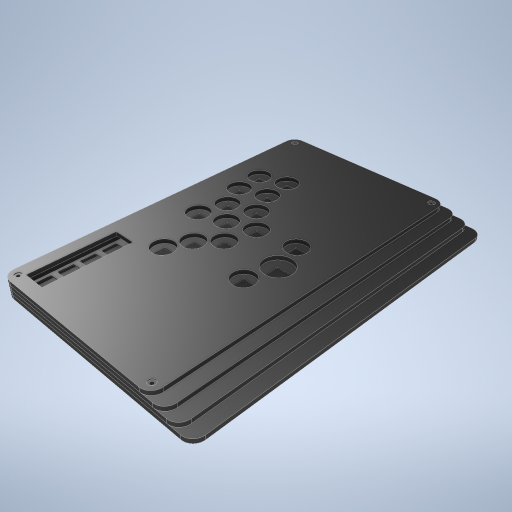
# Autodesk Inventor part: frame
Saved by Autodesk Inventor 2024 (Build 280153000, 153)
## iProperties
Created: 2023-10-17
Part Number: frame
Material: 玻璃
Document SubType Name: Modeling
Designer: Administrator
Density: 2.18 g/cm^3
Appearance: 有光泽 - 黑色
Author: Administrator
Autodesk Inventor part; units mm, degrees
ref_plane "YZ Plane" through (0, 0, 0) normal (1, 0, 0) x (0, 1, 0)
ref_plane "XY Plane" through (0, 0, 0) normal (0, 0, 1) x (1, 0, 0)
ref_plane "底层" through (0, -2, 0) normal (0, 1, 0) x (-1, 0, 0)
ref_plane "第二层" through (0, 4, 0) normal (0, 1, 0) x (-1, 0, 0)
ref_plane "第三层" through (0, 8, 0) normal (0, 1, 0) x (-1, 0, 0)
ref_plane "第四层" through (0, 12, 0) normal (0, 1, 0) x (-1, 0, 0)
sketch "第一层草图" plane through (0, 0, 0) normal (0, 1, 0) x (-1, 0, 0)
  line L0 (90, 150) -> (-90, 150)
  line L1 (-100, 140) -> (-100, -140)
  line L2 (-90, -150) -> (90, -150)
  line L3 (100, -140) -> (100, 140)
  line L4 (100, 150) -> (-100, -150) construction
  line L5 (-100, 150) -> (100, -150) construction
  arc A0 (100, 140) -> (90, 150) centre (90, 140) ccw
  arc A1 (-90, 150) -> (-100, 140) centre (-90, 140) ccw
  arc A2 (-100, -140) -> (-90, -150) centre (-90, -140) ccw
  arc A3 (90, -150) -> (100, -140) centre (90, -140) ccw
  point P0 (0, 0)
  dimension "d2" = 200
  dimension "d3" = 300
  dimension "d4" = 10
  constraints: 12 end point, 8 point on circle, 8 point on line, 8 tangent, 4 centre point, 3 equal radius, 2 midpoint, 2 parallel, 1 horizontal, 1 perpendicular
  measures "d2" distance of L5.end L4.end
  measures "d3" distance of L4.end L5.start
  measures "d4" radius of A0
sketch "第二层草图" plane through (0, 4, 0) normal (0, 1, 0) x (-1, 0, 0)
  line L0 (100, -140) -> (100, 140) projected
  line L1 (100, 0) -> (-88, 0)
  line L2 (90, 150) -> (-78, 150)
  line L3 (-88, 140) -> (-88, -140)
  line L4 (-78, -150) -> (90, -150)
  line L5 (100, -140) -> (100, 140)
  line L6 (100, 150) -> (-88, -150) construction
  line L7 (-88, 150) -> (100, -150) construction
  arc A0 (100, 140) -> (90, 150) centre (90, 140) ccw
  arc A1 (-78, 150) -> (-88, 140) centre (-78, 140) ccw
  arc A2 (-88, -140) -> (-78, -150) centre (-78, -140) ccw
  arc A3 (90, -150) -> (100, -140) centre (90, -140) ccw
  point P0 (0, 0)
  point P1 (6, 0)
  dimension "d101" = 188
  dimension "d102" = 188
  dimension "d103" = 300
  dimension "d104" = 10
  dimension "d125" = 10
  constraints: 14 end point, 8 point on circle, 8 point on line, 8 tangent, 4 centre point, 4 midpoint, 2 equal radius, 2 horizontal, 2 parallel, 1 perpendicular
  measures "d101" distance of L1.start L1.end
  measures "d102" distance of L7.end L6.end
  measures "d103" distance of L6.end L7.start
  measures "d104" radius of A0
  measures "d125" radius of A3
sketch "第三层草图" plane through (0, 8, 0) normal (0, 1, 0) x (-1, 0, 0)
  line L0 (100, -140) -> (100, 140) projected
  line L1 (100, 0) -> (-76, 0)
  line L2 (90, 150) -> (-66, 150)
  line L3 (-76, 140) -> (-76, -140)
  line L4 (-66, -150) -> (90, -150)
  line L5 (100, -140) -> (100, 140)
  line L6 (100, 150) -> (-76, -150) construction
  line L7 (-76, 150) -> (100, -150) construction
  arc A0 (100, 140) -> (90, 150) centre (90, 140) ccw
  arc A1 (-66, 150) -> (-76, 140) centre (-66, 140) ccw
  arc A2 (-76, -140) -> (-66, -150) centre (-66, -140) ccw
  arc A3 (90, -150) -> (100, -140) centre (90, -140) ccw
  point P0 (0, 0)
  point P1 (12, 0)
  dimension "d105" = 176
  dimension "d106" = 176
  dimension "d107" = 300
  dimension "d108" = 10
  constraints: 14 end point, 8 point on circle, 8 point on line, 8 tangent, 4 centre point, 4 midpoint, 3 equal radius, 2 horizontal, 2 parallel, 1 perpendicular
  measures "d105" distance of L1.start L1.end
  measures "d106" distance of L7.end L6.end
  measures "d107" distance of L6.end L7.start
  measures "d108" radius of A0
sketch "第四层草图" plane through (0, 12, 0) normal (0, 1, 0) x (-1, 0, 0)
  line L0 (100, -140) -> (100, 140) projected
  line L1 (100, 0) -> (-64, 0)
  line L2 (90, 150) -> (-54, 150)
  line L3 (-64, 140) -> (-64, -140)
  line L4 (-54, -150) -> (90, -150)
  line L5 (100, -140) -> (100, 140)
  line L6 (100, 150) -> (-64, -150) construction
  line L7 (-64, 150) -> (100, -150) construction
  arc A0 (100, 140) -> (90, 150) centre (90, 140) ccw
  arc A1 (-54, 150) -> (-64, 140) centre (-54, 140) ccw
  arc A2 (-64, -140) -> (-54, -150) centre (-54, -140) ccw
  arc A3 (90, -150) -> (100, -140) centre (90, -140) ccw
  point P0 (0, 0)
  point P1 (18, 0)
  dimension "d109" = 164
  dimension "d110" = 164
  dimension "d111" = 300
  dimension "d112" = 10
  dimension "d113" = 10
  constraints: 14 end point, 8 point on circle, 8 point on line, 8 tangent, 4 centre point, 4 midpoint, 2 equal radius, 2 horizontal, 2 parallel, 1 perpendicular
  measures "d109" distance of L1.start L1.end
  measures "d110" distance of L7.end L6.end
  measures "d111" distance of L6.end L7.start
  measures "d112" radius of A0
  measures "d113" radius of A2
sketch "底层草图" plane through (0, -2, 0) normal (0, 1, 0) x (-1, 0, 0)
  line L0 (98, 140) -> (98, -140)
  arc A0 (90, -148) -> (98, -140) centre (90, -140) ccw
  line L1 (90, -148) -> (-90, -148)
  arc A1 (-98, -140) -> (-90, -148) centre (-90, -140) ccw
  line L2 (-98, -140) -> (-98, 140)
  arc A2 (-90, 148) -> (-98, 140) centre (-90, 140) ccw
  line L3 (-90, 148) -> (90, 148)
  arc A3 (98, 140) -> (90, 148) centre (90, 140) ccw
  point P0 (0, 0)
  constraints: 8 end point, 8 point on circle, 4 centre point
extrude "拉伸25" add sketch "底层草图" along normal blind 2
extrude "拉伸26" add sketch "第一层草图" along normal blind 4 separate body
extrude "拉伸27" add sketch "第二层草图" along normal blind 4 separate body
extrude "拉伸28" add sketch "第三层草图" along normal blind 4 separate body
extrude "拉伸29" add sketch "第四层草图" along normal blind 4 separate body
sketch "草图20" plane through (0, 16, 0) normal (0, 1, 0) x (1, 0, 0)
  line L0 (-100, 140) -> (-100, -140) projected
  arc A0 (-100, -140) -> (-90, -150) centre (-90, -140) ccw projected
  line L1 (-90, -150) -> (54, -150) projected
  arc A1 (54, -150) -> (64, -140) centre (54, -140) ccw projected
  line L2 (64, -140) -> (64, 140) projected
  arc A2 (64, 140) -> (54, 150) centre (54, 140) ccw projected
  line L3 (54, 150) -> (-90, 150) projected
  arc A3 (-90, 150) -> (-100, 140) centre (-90, 140) ccw projected
  line L4 (-90, -140) -> (-92.1213, -142.1213)
  line L5 (-90, -140) -> (-87, -140) construction
  circle A4 centre (-92.1213, -142.1213) radius 2.75
  line L6 (-90, 140) -> (-92.1213, 142.1213)
  circle A5 centre (-92.1213, 142.1213) radius 2.75
  line L7 (54, -140) -> (56.1213, -142.1213)
  line L8 (54, -140) -> (57, -140) construction
  circle A6 centre (56.1213, -142.1213) radius 2.75
  line L9 (54, 140) -> (56.1213, 142.1213)
  circle A7 centre (56.1213, 142.1213) radius 2.75
  line L10 (-88, -138) -> (-88, 138)
  line L11 (-88, 138) -> (52, 138)
  line L12 (52, 138) -> (52, -138)
  line L13 (52, -138) -> (-88, -138)
  line L14 (-89.3713, -142.1213) -> (-90.7463, -144.5029)
  line L15 (-90.7463, -144.5029) -> (-93.4963, -144.5029)
  line L16 (-93.4963, -144.5029) -> (-94.8713, -142.1213)
  line L17 (-94.8713, -142.1213) -> (-93.4963, -139.7398)
  line L18 (-93.4963, -139.7398) -> (-90.7463, -139.7398)
  line L19 (-90.7463, -139.7398) -> (-89.3713, -142.1213)
  line L20 (-89.3713, 142.1213) -> (-90.7463, 139.7398)
  line L21 (-90.7463, 139.7398) -> (-93.4963, 139.7398)
  line L22 (-93.4963, 139.7398) -> (-94.8713, 142.1213)
  line L23 (-94.8713, 142.1213) -> (-93.4963, 144.5029)
  line L24 (-93.4963, 144.5029) -> (-90.7463, 144.5029)
  line L25 (-90.7463, 144.5029) -> (-89.3713, 142.1213)
  line L26 (58.8713, 142.1213) -> (57.4963, 139.7398)
  line L27 (57.4963, 139.7398) -> (54.7463, 139.7398)
  line L28 (54.7463, 139.7398) -> (53.3713, 142.1213)
  line L29 (53.3713, 142.1213) -> (54.7463, 144.5029)
  line L30 (54.7463, 144.5029) -> (57.4963, 144.5029)
  line L31 (57.4963, 144.5029) -> (58.8713, 142.1213)
  line L32 (58.8713, -142.1213) -> (57.4963, -144.5029)
  line L33 (57.4963, -144.5029) -> (54.7463, -144.5029)
  line L34 (54.7463, -144.5029) -> (53.3713, -142.1213)
  line L35 (53.3713, -142.1213) -> (54.7463, -139.7398)
  line L36 (54.7463, -139.7398) -> (57.4963, -139.7398)
  line L37 (57.4963, -139.7398) -> (58.8713, -142.1213)
  circle A8 centre (-92.1213, -142.1213) radius 1.6
  circle A9 centre (-92.1213, 142.1213) radius 1.6
  circle A10 centre (56.1213, -142.1213) radius 1.6
  circle A11 centre (56.1213, 142.1213) radius 1.6
  point P0 (0, 0)
  dimension "d128" = 5.5
  dimension "d130" = 5.5
  dimension "d132" = 5.5
  dimension "d134" = 5.5
  dimension "d126" = 3
  dimension "d127" = 135
  dimension "d129" = 3
  dimension "d131" = 45
  dimension "d133" = 3
  dimension "d135" = 12
  dimension "d136" = 3.2
  dimension "d137" = 3.2
  dimension "d138" = 3.2
  dimension "d139" = 3.2
  constraints: 68 end point, 12 coincident, 4 centre point, 4 horizontal alignment, 2 equal length, 2 horizontal, 63 other
  measures "d126" distance of L4.start L4.end
  measures "d127" angle of L4 L5
  measures "d129" distance of L6.start L6.end
  measures "d131" angle of L7 L8
  measures "d133" distance of L9.start L9.end
  measures "d135" distance between parallel lines of L0 L10
  measures "d136" diameter of A8
  measures "d137" diameter of A9
  measures "d138" diameter of A10
  measures "d139" diameter of A11
extrude "拉伸30" cut sketch "草图20" against normal up to surface (18 mm away) contours L10 L11 L12 L13 bodies 4 3 2
hole "四角固定孔" at (-92.1213, 16, 142.1213) at (-92.1213, 16, -142.1213) at (56.1213, 16, -142.1213) at (56.1213, 16, 142.1213) direction (0, -1, 0) diameter 3.2 end through all counterbore diameter 6.2 counterbore depth 1 bodies 5
extrude "六角通孔1" cut sketch "草图20" against normal through all contours L19 L14 L15 L16 L17 L18 | A8 bodies 4 3 2
extrude "六角通孔2" cut sketch "草图20" against normal through all contours L35 L36 L37 L32 L33 L34 | A10 bodies 4 3 2
extrude "六角通孔3" cut sketch "草图20" against normal through all contours L28 L29 L30 L31 L26 L27 | A11 bodies 4 3 2
extrude "六角通孔4" cut sketch "草图20" against normal through all contours L20 L21 L22 L23 L24 L25 | A9 bodies 4 3 2
sketch "第二层开孔草图" plane through (0, 8, 0) normal (0, 1, 0) x (1, 0, 0)
  line L0 (-100, 0) -> (-98, 0)
  line L1 (-100, 0) -> (-98, 0) construction
  line L2 (-98, 0) -> (-88, 0)
  line L3 (-98, -15) -> (-88, -15)
  line L4 (-88, -15) -> (-88, 15)
  line L5 (-88, 15) -> (-98, 15)
  line L6 (-98, 15) -> (-98, -15)
  line L7 (-98, -15) -> (-88, 15) construction
  line L8 (-88, -15) -> (-98, 15) construction
  line L9 (-100, -4.9) -> (-98, -4.9)
  line L10 (-98, -4.9) -> (-98, 4.9)
  line L11 (-98, 4.9) -> (-100, 4.9)
  line L12 (-100, 4.9) -> (-100, -4.9)
  line L13 (-100, -4.9) -> (-98, 4.9) construction
  line L14 (-98, -4.9) -> (-100, 4.9) construction
  line L15 (-88, 76.5) -> (-98, 76.5)
  line L16 (-98, 76.5) -> (-100, 76.5)
  line L17 (-98, 76.5) -> (-96, 76.5) construction
  line L18 (-98, 61.5) -> (-88, 61.5)
  line L19 (-88, 61.5) -> (-88, 91.5)
  line L20 (-88, 91.5) -> (-98, 91.5)
  line L21 (-98, 91.5) -> (-98, 61.5)
  line L22 (-98, 61.5) -> (-88, 91.5) construction
  line L23 (-88, 61.5) -> (-98, 91.5) construction
  line L24 (-100, 71.6) -> (-98, 71.6)
  line L25 (-98, 71.6) -> (-98, 81.4)
  line L26 (-98, 81.4) -> (-100, 81.4)
  line L27 (-100, 81.4) -> (-100, 71.6)
  line L28 (-100, 71.6) -> (-98, 81.4) construction
  line L29 (-98, 71.6) -> (-100, 81.4) construction
  line L30 (-88, 15) -> (-88, 61.5)
  line L31 (-88, 38.25) -> (-100, 38.25)
  line L32 (-100, 26.75) -> (-88, 26.75)
  line L33 (-88, 26.75) -> (-88, 49.75)
  line L34 (-88, 49.75) -> (-100, 49.75)
  line L35 (-100, 49.75) -> (-100, 26.75)
  line L36 (-100, 26.75) -> (-88, 49.75) construction
  line L37 (-88, 26.75) -> (-100, 49.75) construction
  line L38 (-91.2527, 26.75) -> (-92.6263, 24.3708)
  line L39 (-92.6263, 24.3708) -> (-95.3737, 24.3708)
  line L40 (-95.3737, 24.3708) -> (-96.7473, 26.75)
  line L41 (-96.7473, 26.75) -> (-95.3737, 29.1292)
  line L42 (-95.3737, 29.1292) -> (-92.6263, 29.1292)
  line L43 (-92.6263, 29.1292) -> (-91.2527, 26.75)
  line L44 (-91.2527, 49.75) -> (-92.6263, 47.3708)
  line L45 (-92.6263, 47.3708) -> (-95.3737, 47.3708)
  line L46 (-95.3737, 47.3708) -> (-96.7473, 49.75)
  line L47 (-96.7473, 49.75) -> (-95.3737, 52.1292)
  line L48 (-95.3737, 52.1292) -> (-92.6263, 52.1292)
  line L49 (-92.6263, 52.1292) -> (-91.2527, 49.75)
  line L50 (-88, -15) -> (-88, -26.75)
  line L51 (-88, -26.75) -> (-100, -26.75)
  line L52 (-88, 91.5) -> (-88, 103.25)
  line L53 (-88, 103.25) -> (-100, 103.25)
  line L54 (-91.2501, -26.75) -> (-92.625, -29.1315)
  line L55 (-92.625, -29.1315) -> (-95.375, -29.1315)
  line L56 (-95.375, -29.1315) -> (-96.7499, -26.75)
  line L57 (-96.7499, -26.75) -> (-95.375, -24.3685)
  line L58 (-95.375, -24.3685) -> (-92.625, -24.3685)
  line L59 (-92.625, -24.3685) -> (-91.2501, -26.75)
  line L60 (-91.2501, 103.25) -> (-92.625, 100.8685)
  line L61 (-92.625, 100.8685) -> (-95.375, 100.8685)
  line L62 (-95.375, 100.8685) -> (-96.7499, 103.25)
  line L63 (-96.7499, 103.25) -> (-95.375, 105.6315)
  line L64 (-95.375, 105.6315) -> (-92.625, 105.6315)
  line L65 (-92.625, 105.6315) -> (-91.2501, 103.25)
  point P0 (0, 0)
  point P1 (-93, 0)
  point P2 (-99, 0)
  point P3 (-93, 76.5)
  point P4 (-99, 76.5)
  point P5 (-94, 38.25)
  point P6 (-94, 26.75)
  point P7 (-94, 49.75)
  point P8 (-94, -26.75)
  point P9 (-94, 103.25)
  dimension "d164" = 2
  dimension "d165" = 0
  dimension "d166" = 30
  dimension "d167" = 9.8
  dimension "d172" = 10
  dimension "d173" = 2
  dimension "d174" = 180
  dimension "d175" = 10
  dimension "d176" = 30
  dimension "d177" = 2
  dimension "d178" = 9.8
  dimension "d183" = 23
  dimension "d189" = 11.75
  dimension "d190" = 11.75
  constraints: 132 end point, 10 midpoint, 2 collinear, 2 horizontal, 52 other
  measures "d164" distance of L0.start L0.end
  measures "d165" distance between parallel lines of L0 L1
  measures "d166" distance of L4.end L3.end
  measures "d167" distance of L10.end L9.end
  measures "d172" distance of L15.start L15.end
  measures "d173" distance of L16.start L16.end
  measures "d174" angle of L16 L17
  measures "d175" distance of L20.end L19.end
  measures "d176" distance of L19.end L18.end
  measures "d177" distance of L26.end L25.end
  measures "d178" distance of L25.end L24.end
  measures "d183" distance of L33.end L32.end
  measures "d189" distance of L50.start L50.end
  measures "d190" distance of L52.start L52.end
extrude "拉伸35" cut sketch "第二层开孔草图" against normal blind 10 contours L6 L5 L4 L2 | L2 L4 L3 L6 bodies 3 2
extrude "拉伸36" cut sketch "第二层开孔草图" against normal blind 10 contours L12 L11 L6 L0 | L0 L6 L9 L12 bodies 3
extrude "拉伸37" cut sketch "第二层开孔草图" against normal through all contours L19 L18 L21 L15 | L15 L21 L20 L19 bodies 3 2
extrude "拉伸38" cut sketch "第二层开孔草图" against normal through all contours L21 L24 L27 L16 | L16 L27 L26 L21 bodies 3
ref_plane "第三层开孔面" through (0, 12, 0) normal (0, 1, 0) x (1, 0, 0)
sketch "第三层开孔草图" plane through (0, 12, 0) normal (0, 1, 0) x (1, 0, 0)
  line L0 (-95.3737, 29.1292) -> (-92.6263, 29.1292) projected
  line L1 (-96.7473, 26.75) -> (-95.3737, 29.1292) projected
  line L2 (-95.3737, 24.3708) -> (-96.7473, 26.75) projected
  line L3 (-92.6263, 24.3708) -> (-95.3737, 24.3708) projected
  line L4 (-91.2527, 26.75) -> (-92.6263, 24.3708) projected
  line L5 (-92.6263, 29.1292) -> (-91.2527, 26.75) projected
  line L6 (-91.2527, 49.75) -> (-92.6263, 47.3708) projected
  line L7 (-92.6263, 47.3708) -> (-95.3737, 47.3708) projected
  line L8 (-95.3737, 47.3708) -> (-96.7473, 49.75) projected
  line L9 (-96.7473, 49.75) -> (-95.3737, 52.1292) projected
  line L10 (-95.3737, 52.1292) -> (-92.6263, 52.1292) projected
  line L11 (-92.6263, 52.1292) -> (-91.2527, 49.75) projected
  line L12 (-96.7499, -26.75) -> (-95.375, -24.3685) projected
  line L13 (-95.375, -29.1315) -> (-96.7499, -26.75) projected
  line L14 (-92.625, -29.1315) -> (-95.375, -29.1315) projected
  line L15 (-91.2501, -26.75) -> (-92.625, -29.1315) projected
  line L16 (-92.625, -24.3685) -> (-91.2501, -26.75) projected
  line L17 (-95.375, -24.3685) -> (-92.625, -24.3685) projected
  line L18 (-95.375, 100.8685) -> (-96.7499, 103.25) projected
  line L19 (-92.625, 100.8685) -> (-95.375, 100.8685) projected
  line L20 (-91.2501, 103.25) -> (-92.625, 100.8685) projected
  line L21 (-92.625, 105.6315) -> (-91.2501, 103.25) projected
  line L22 (-95.375, 105.6315) -> (-92.625, 105.6315) projected
  line L23 (-96.7499, 103.25) -> (-95.375, 105.6315) projected
  point P0 (0, 0)
extrude "中间层固定孔" cut sketch "第三层开孔草图" against normal through all bodies 4 3 2
sketch "底部孔草图" plane through (0, -2, 0) normal (0, -1, 0) x (1, 0, 0)
  circle A0 centre (-92.1213, -142.1213) radius 2.75 projected
  circle A1 centre (56.1213, -142.1213) radius 2.75 projected
  circle A2 centre (56.1213, 142.1213) radius 2.75 projected
  circle A3 centre (-92.1213, 142.1213) radius 2.75 projected
  line L0 (-96.7473, -26.75) -> (-95.3737, -24.3708) projected
  line L1 (-95.3737, -29.1292) -> (-96.7473, -26.75) projected
  line L2 (-92.6263, -29.1292) -> (-95.3737, -29.1292) projected
  line L3 (-91.2527, -26.75) -> (-92.6263, -29.1292) projected
  line L4 (-92.6263, -24.3708) -> (-91.2527, -26.75) projected
  line L5 (-95.3737, -24.3708) -> (-92.6263, -24.3708) projected
  line L6 (-95.375, 24.3685) -> (-96.7499, 26.75) projected
  line L7 (-96.7499, 26.75) -> (-95.375, 29.1315) projected
  line L8 (-95.375, 29.1315) -> (-92.625, 29.1315) projected
  line L9 (-92.625, 29.1315) -> (-91.2501, 26.75) projected
  line L10 (-91.2501, 26.75) -> (-92.625, 24.3685) projected
  line L11 (-92.625, 24.3685) -> (-95.375, 24.3685) projected
  circle A4 centre (-94, -26.75) radius 2.3792
  circle A5 centre (-94, 26.75) radius 2.3815
  point P0 (0, 0)
  constraints: 6 tangent, 2 centre point
hole "底板定位孔" at (-92.1213, -2, -142.1213) at (-92.1213, -2, 142.1213) at (56.1213, -2, 142.1213) at (56.1213, -2, -142.1213) at (-94, -2, -26.75) at (-94, -2, 26.75) direction (0, 1, 0) diameter 3.2 end through all counterbore diameter 6.6 counterbore depth 1 bodies 1
ref_plane "按键孔位平面" through (0, 16, 0) normal (0, 1, 0) x (1, 0, 0)
sketch "按键孔位图" plane through (0, 16, 0) normal (0, 1, 0) x (1, 0, 0)
  circle A0 centre (-65.0378, 1.142) radius 10.5
  circle A1 centre (-58.3085, 26.2561) radius 10.5
  circle A2 centre (-39.9237, 7.8713) radius 10.5
  line L0 (-39.9237, 7.8713) -> (-39.9237, 33.8713)
  line L1 (-21.2884, -11.7513) -> (-21.2884, 10.2487)
  line L2 (-39.9237, 7.8713) -> (-58.3085, 26.2561)
  line L3 (-58.3085, 26.2561) -> (-69.2965, 49.8201)
  line L4 (-69.2965, 49.8201) -> (-71.5626, 75.7211)
  circle A3 centre (-37.5518, -28.0147) radius 10.5
  line L5 (-15.2859, 15.7913) -> (-33.6707, 34.176)
  line L6 (-33.6707, 34.176) -> (-44.6587, 57.74)
  line L7 (-44.6587, 57.74) -> (-46.9248, 83.6411)
  circle A4 centre (-21.2884, -11.7513) radius 10.5
  circle A5 centre (-69.2965, 49.8201) radius 10.5
  circle A6 centre (-33.6707, 34.176) radius 10.5
  line L8 (-15.2859, 15.7913) -> (-15.2859, 41.7913)
  circle A7 centre (-15.2859, 15.7913) radius 10.5
  circle A8 centre (-47.2721, -48.8598) radius 10.5
  circle A9 centre (-44.6587, 57.74) radius 10.5
  circle A10 centre (-71.5626, 75.7211) radius 10.5
  circle A11 centre (-46.9248, 83.6411) radius 10.5
  circle A12 centre (21.9427, 20.1213) radius 10.5
  circle A13 centre (21.9427, -33.997) radius 10.5
  circle A14 centre (29.1401, -6.9379) radius 13.5
  line L9 (-88, -138) -> (-88, -128)
  line L10 (-88, -128) -> (-78, -128)
  line L11 (-88, -128) -> (-78, -128) construction
  line L12 (-68.85, -137.15) -> (-68.85, -118.85)
  line L13 (-68.85, -118.85) -> (-87.15, -118.85)
  line L14 (-87.15, -118.85) -> (-87.15, -137.15)
  line L15 (-87.15, -137.15) -> (-68.85, -118.85) construction
  line L16 (-68.85, -137.15) -> (-87.15, -118.85) construction
  line L17 (-78, -128) -> (-78, -109)
  line L18 (-78, -109) -> (-78, -90)
  line L19 (-78, -90) -> (-78, -71)
  line L20 (-87.15, -118.15) -> (-68.85, -118.15)
  line L21 (-68.85, -118.15) -> (-68.85, -99.85)
  line L22 (-68.85, -99.85) -> (-87.15, -99.85)
  line L23 (-87.15, -99.85) -> (-87.15, -118.15)
  line L24 (-87.15, -118.15) -> (-68.85, -99.85) construction
  line L25 (-68.85, -118.15) -> (-87.15, -99.85) construction
  line L26 (-87.15, -99.15) -> (-68.85, -99.15)
  line L27 (-68.85, -99.15) -> (-68.85, -80.85)
  line L28 (-68.85, -80.85) -> (-87.15, -80.85)
  line L29 (-87.15, -80.85) -> (-87.15, -99.15)
  line L30 (-87.15, -99.15) -> (-68.85, -80.85) construction
  line L31 (-68.85, -99.15) -> (-87.15, -80.85) construction
  line L32 (-87.15, -80.15) -> (-68.85, -80.15)
  line L33 (-68.85, -80.15) -> (-68.85, -61.85)
  line L34 (-87.15, -61.85) -> (-87.15, -80.15)
  line L35 (-87.15, -80.15) -> (-68.85, -61.85) construction
  line L36 (-68.85, -80.15) -> (-87.15, -61.85) construction
  line L37 (-87.15, -137.15) -> (-68.85, -137.15)
  line L38 (-68.85, -61.85) -> (-87.15, -61.85)
  line L39 (-67.85, -60.85) -> (-67.85, -138.15)
  line L40 (-67.85, -138.15) -> (-88.15, -138.15)
  line L41 (-88.15, -138.15) -> (-88.15, -60.85)
  line L42 (-88.15, -60.85) -> (-67.85, -60.85)
  line L43 (-100, 140) -> (-100, -140) projected
  arc A15 (-100, -140) -> (-90, -150) centre (-90, -140) ccw projected
  line L44 (-90, -150) -> (54, -150) projected
  arc A16 (54, -150) -> (64, -140) centre (54, -140) ccw projected
  line L45 (64, -140) -> (64, 140) projected
  arc A17 (64, 140) -> (54, 150) centre (54, 140) ccw projected
  line L46 (54, 150) -> (-90, 150) projected
  arc A18 (-90, 150) -> (-100, 140) centre (-90, 140) ccw projected
  line L47 (-21.2884, -11.7513) -> (-37.5518, -28.0147)
  line L48 (-21.2884, -11.7513) -> (1.7116, -11.7513) construction
  line L49 (-37.5518, -28.0147) -> (-47.2721, -48.8598)
  line L50 (-37.5518, -28.0147) -> (-14.5518, -28.0147) construction
  line L51 (-57.8511, -135.3115) -> (-24.3511, -135.3115)
  line L52 (-24.3511, -135.3115) -> (-24.3511, -99.9115)
  line L53 (-24.3511, -99.9115) -> (-57.8511, -99.9115)
  line L54 (-57.8511, -99.9115) -> (-57.8511, -135.3115)
  line L55 (-57.8511, -117.6115) -> (-51.5011, -117.6115)
  line L56 (-51.5011, -117.6115) -> (-34.8011, -117.6115)
  line L57 (-51.5011, -133.3215) -> (-34.8011, -133.3215)
  line L58 (-34.8011, -133.3215) -> (-34.8011, -101.9015)
  line L59 (-34.8011, -101.9015) -> (-51.5011, -101.9015)
  line L60 (-51.5011, -101.9015) -> (-51.5011, -133.3215)
  line L61 (-51.5011, -133.3215) -> (-34.8011, -101.9015) construction
  line L62 (-34.8011, -133.3215) -> (-51.5011, -101.9015) construction
  line L63 (-24.3511, -135.3115) -> (-26.8511, -135.3115)
  line L64 (-26.8511, -135.3115) -> (-26.8511, -132.7115)
  line L65 (-26.8511, -132.7115) -> (-24.3511, -132.7115)
  line L66 (-24.3511, -132.7115) -> (-24.3511, -135.3115)
  line L67 (-24.3511, -99.9115) -> (-26.8511, -99.9115)
  line L68 (-26.8511, -99.9115) -> (-26.8511, -102.5115)
  line L69 (-26.8511, -102.5115) -> (-24.3511, -102.5115)
  line L70 (-24.3511, -102.5115) -> (-24.3511, -99.9115)
  line L71 (-57.8511, -135.3115) -> (-55.3511, -135.3115)
  line L72 (-55.3511, -135.3115) -> (-55.3511, -132.7115)
  line L73 (-55.3511, -132.7115) -> (-57.8511, -132.7115)
  line L74 (-57.8511, -132.7115) -> (-57.8511, -135.3115)
  line L75 (-57.8511, -99.9115) -> (-55.3511, -99.9115)
  line L76 (-55.3511, -99.9115) -> (-55.3511, -102.5115)
  line L77 (-55.3511, -102.5115) -> (-57.8511, -102.5115)
  line L78 (-57.8511, -102.5115) -> (-57.8511, -99.9115)
  circle A19 centre (-55.3511, -132.7115) radius 1.5
  circle A20 centre (-55.3511, -102.5115) radius 1.5
  circle A21 centre (-26.8511, -102.5115) radius 1.5
  circle A22 centre (-26.8511, -132.7115) radius 1.5
  line L79 (-51.4261, -129.1115) -> (-57.9261, -129.1115)
  line L80 (-57.9261, -129.1115) -> (-57.9261, -106.1115)
  line L81 (-57.9261, -106.1115) -> (-51.4261, -106.1115)
  line L82 (-51.4261, -106.1115) -> (-51.4261, -129.1115)
  line L83 (-51.4261, -129.1115) -> (-57.9261, -106.1115) construction
  line L84 (-57.9261, -129.1115) -> (-51.4261, -106.1115) construction
  point P0 (0, 0)
  point P1 (-41.7048, -37.7302)
  point P2 (-38.4537, -38.6945)
  point P3 (-29.4201, -19.883)
  point P4 (-31.4383, -17.1578)
  point P5 (-43.1511, -117.6115)
  point P6 (-54.6761, -117.6115)
  dimension "d195" = 10
  dimension "d196" = 10
  dimension "d197" = 0
  dimension "d198" = 18.3
  dimension "d199" = 18.3
  dimension "d200" = 19
  dimension "d202" = 19
  dimension "d203" = 19
  dimension "d204" = 18.3
  dimension "d205" = 18.3
  dimension "d206" = 18.3
  dimension "d207" = 18.3
  dimension "d208" = 18.3
  dimension "d209" = 18.3
  dimension "d268" = 21
  dimension "d269" = 21
  dimension "d270" = 21
  dimension "d271" = 21
  dimension "d272" = 27
  dimension "d273" = 21
  dimension "d274" = 21
  dimension "d275" = 21
  dimension "d276" = 21
  dimension "d277" = 21
  dimension "d278" = 21
  dimension "d279" = 21
  dimension "d280" = 21
  dimension "d281" = 21
  dimension "d282" = 21
  dimension "d283" = 23
  dimension "d284" = 135
  dimension "d285" = 23
  dimension "d286" = 115
  dimension "d288" = 33.5
  dimension "d289" = 35.4
  dimension "d290" = 6.35
  dimension "d291" = 16.7
  dimension "d292" = 16.7
  dimension "d293" = 31.42
  dimension "d294" = 2.5
  dimension "d295" = 2.6
  dimension "d296" = 2.5
  dimension "d297" = 2.6
  dimension "d298" = 2.5
  dimension "d299" = 2.6
  dimension "d300" = 2.5
  dimension "d301" = 2.6
  dimension "d302" = 3
  dimension "d303" = 3
  dimension "d304" = 3
  dimension "d305" = 3
  dimension "d306" = 6.5
  dimension "d307" = 23
  constraints: 162 end point, 19 centre point, 12 midpoint, 3 equal length, 3 horizontal
  measures "d195" distance of L9.start L9.end
  measures "d196" distance of L10.start L10.end
  measures "d197" distance between parallel lines of L10 L11
  measures "d198" distance of L13.end L12.end
  measures "d199" distance of L12.end L12.start
  measures "d200" distance of L17.start L17.end
  measures "d202" distance of L18.start L18.end
  measures "d203" distance of L19.start L19.end
  measures "d204" distance of L22.end L21.end
  measures "d205" distance of L21.end L20.end
  measures "d206" distance of L28.end L27.end
  measures "d207" distance of L27.end L26.end
  measures "d208" distance of L34.start L33.end
  measures "d209" distance of L33.end L32.end
  measures "d268" diameter of A8
  measures "d269" diameter of A3
  measures "d270" diameter of A4
  measures "d271" diameter of A13
  measures "d272" diameter of A14
  measures "d273" diameter of A12
  measures "d274" diameter of A7
  measures "d275" diameter of A2
  measures "d276" diameter of A1
  measures "d277" diameter of A0
  measures "d278" diameter of A6
  measures "d279" diameter of A9
  measures "d280" diameter of A5
  measures "d281" diameter of A10
  measures "d282" diameter of A11
  measures "d283" distance of L47.start L47.end
  measures "d284" angle of L47 L48
  measures "d285" distance of L49.start L49.end
  measures "d286" angle of L49 L50
  measures "d288" distance of L53.end L52.end
  measures "d289" distance of L52.end L51.end
  measures "d290" distance of L55.start L55.end
  measures "d291" distance of L56.start L56.end
  measures "d292" distance of L59.end L58.end
  measures "d293" distance of L58.end L57.end
  measures "d294" distance of L64.end L65.end
  measures "d295" distance of L63.end L64.end
  measures "d296" distance of L69.end L68.end
  measures "d297" distance of L68.end L67.end
  measures "d298" distance of L73.end L72.end
  measures "d299" distance of L72.end L71.end
  measures "d300" distance of L76.end L77.end
  measures "d301" distance of L75.end L76.end
  measures "d302" diameter of A19
  measures "d303" diameter of A20
  measures "d304" diameter of A21
  measures "d305" diameter of A22
  measures "d306" distance of L80.end L81.end
  measures "d307" distance of L79.end L80.end
extrude "按键开孔" cut sketch "按键孔位图" against normal through all contours A0 | A1 L2 L3 | L3 L2 A1 | A2 L2 L0 | L0 L2 A2 | L47 A4 L1 | L1 A4 L47 | A5 L4 L3 | L3 L4 A5 | A3 L49 L47 | L47 L49 A3 | L8 A7 L5 | L5 A7 L8 | A6 L6 L5 | L5 L6 A6 | A9 L7 L6 | L6 L7 A9 | A8 | A10 | A11 | A12 | A13 | A14 | L14 L13 L17 L10 | L10 L17 L13 L12 L37 L14 | L20 L23 L22 L18 L17 | L17 L18 L22 L21 L20 | L26 L29 L28 L19 L18 | L18 L19 L28 L27 L26 | L34 L38 L33 L32 | L39 L40 L41 L42 bodies 5
ref_plane "PCB平面" through (0, 3.5, 0) normal (0, 1, 0) x (1, 0, 0)
sketch "PCB草图" plane through (0, 3.5, 0) normal (0, 1, 0) x (1, 0, 0)
  line L0 (-88, -138) -> (-88, -15) projected
  line L1 (-88, -15) -> (-98, -15) projected
  line L2 (-98, -15) -> (-98, 15) projected
  line L3 (-98, 15) -> (-88, 15) projected
  line L4 (-88, 15) -> (-88, 61.5) projected
  line L5 (-88, 61.5) -> (-98, 61.5) projected
  line L6 (-98, 61.5) -> (-98, 91.5) projected
  line L7 (-98, 91.5) -> (-88, 91.5) projected
  line L8 (-88, 91.5) -> (-88, 138) projected
  line L9 (-88, 138) -> (52, 138) projected
  line L10 (52, 138) -> (52, -138) projected
  line L11 (52, -138) -> (-88, -138) projected
  line L12 (-87.5, -14.5) -> (-87.5, -137.5)
  line L13 (-87.5, -137.5) -> (51.5, -137.5)
  line L14 (51.5, -137.5) -> (51.5, 137.5)
  line L15 (51.5, 137.5) -> (-87.5, 137.5)
  line L16 (-87.5, 137.5) -> (-87.5, 91)
  line L17 (-87.5, 91) -> (-97.5, 91)
  line L18 (-97.5, 91) -> (-97.5, 62)
  line L19 (-97.5, 62) -> (-87.5, 62)
  line L20 (-87.5, 62) -> (-87.5, 14.5)
  line L21 (-87.5, 14.5) -> (-97.5, 14.5)
  line L22 (-97.5, 14.5) -> (-97.5, -14.5)
  line L23 (-97.5, -14.5) -> (-87.5, -14.5)
  line L24 (-87.5, -137.5) -> (-80.4289, -130.4289)
  line L25 (-87.5, -137.5) -> (-77.5, -137.5) construction
  line L26 (51.5, -137.5) -> (44.4289, -130.4289)
  line L27 (51.5, -137.5) -> (61.5, -137.5) construction
  line L28 (51.5, 137.5) -> (44.4289, 130.4289)
  line L29 (51.5, 137.5) -> (61.5, 137.5) construction
  line L30 (-87.5, 137.5) -> (-80.4289, 130.4289)
  line L31 (-87.5, 137.5) -> (-77.5, 137.5) construction
  line L32 (-80.4289, -130.4289) -> (-40.4289, -130.4289)
  line L33 (-80.4289, -130.4289) -> (-40.4289, -130.4289) construction
  line L34 (44.4289, -130.4289) -> (4.4289, -130.4289)
  line L35 (44.4289, -130.4289) -> (84.4289, -130.4289) construction
  line L36 (-80.4289, 130.4289) -> (-40.4289, 130.4289)
  line L37 (-80.4289, 130.4289) -> (-40.4289, 130.4289) construction
  line L38 (44.4289, 130.4289) -> (4.4289, 130.4289)
  line L39 (44.4289, -130.4289) -> (44.4289, -44.4289)
  line L40 (44.4289, -130.4289) -> (130.4289, -130.4289) construction
  line L41 (44.4289, 130.4289) -> (44.4289, 44.4289)
  line L42 (44.4289, 130.4289) -> (130.4289, 130.4289) construction
  line L43 (-97.5, -14.5) -> (-93.9645, -10.9645)
  line L44 (-97.5, 14.5) -> (-93.9645, 10.9645)
  line L45 (-97.5, 62) -> (-93.9645, 65.5355)
  line L46 (-97.5, 91) -> (-93.9645, 87.4645)
  line L47 (-80.4289, -130.4289) -> (-80.4289, -44.4289)
  circle A0 centre (-80.4289, -44.4289) radius 1.5
  circle A1 centre (-40.4289, -130.4289) radius 1.5
  circle A2 centre (4.4289, -130.4289) radius 1.5
  circle A3 centre (44.4289, -44.4289) radius 1.5
  circle A4 centre (44.4289, 44.4289) radius 1.5
  circle A5 centre (4.4289, 130.4289) radius 1.5
  circle A6 centre (-40.4289, 130.4289) radius 1.5
  circle A7 centre (-93.9645, -10.9645) radius 1.5
  circle A8 centre (-93.9645, 10.9645) radius 1.5
  circle A9 centre (-93.9645, 65.5355) radius 1.5
  circle A10 centre (-93.9645, 87.4645) radius 1.5
  line L48 (44.4289, -44.4289) -> (-18.0001, -44.4289)
  line L49 (44.4289, 44.4289) -> (-18.0001, 44.4289)
  circle A11 centre (-18.0001, -44.4289) radius 1.5
  circle A12 centre (-18.0001, 44.4289) radius 1.5
  line L50 (-80.4289, 130.4289) -> (-80.4289, 44.4289)
  circle A13 centre (-80.4289, 44.4289) radius 1.5
  point P0 (0, 0)
  dimension "d214" = 0.5
  dimension "d215" = 10
  dimension "d216" = 45
  dimension "d217" = 10
  dimension "d218" = 135
  dimension "d219" = 10
  dimension "d220" = 135
  dimension "d221" = 10
  dimension "d222" = 45
  dimension "d223" = 40
  dimension "d225" = 40
  dimension "d227" = 40
  dimension "d228" = 0
  dimension "d229" = 40
  dimension "d230" = 86
  dimension "d231" = 90
  dimension "d232" = 86
  dimension "d233" = 90
  dimension "d234" = 5
  dimension "d235" = 5
  dimension "d236" = 5
  dimension "d237" = 5
  dimension "d238" = 86
  dimension "d239" = 3
  dimension "d240" = 3
  dimension "d241" = 3
  dimension "d242" = 3
  dimension "d243" = 3
  dimension "d244" = 3
  dimension "d245" = 3
  dimension "d246" = 3
  dimension "d247" = 3
  dimension "d248" = 3
  dimension "d249" = 3
  dimension "d250" = 62.429
  dimension "d251" = 62.429
  dimension "d252" = 3
  dimension "d253" = 3
  dimension "d257" = 86
  dimension "d258" = 3
  constraints: 78 end point, 14 centre point, 9 equal length, 9 horizontal, 11 other
  measures "d214" distance between parallel lines of L0 L12
  measures "d215" distance of L24.start L24.end
  measures "d216" angle of L25 L24
  measures "d217" distance of L26.start L26.end
  measures "d218" angle of L27 L26
  measures "d219" distance of L28.start L28.end
  measures "d220" angle of L28 L29
  measures "d221" distance of L30.start L30.end
  measures "d222" angle of L30 L31
  measures "d223" distance of L32.start L32.end
  measures "d225" distance of L34.start L34.end
  measures "d227" distance of L36.start L36.end
  measures "d228" distance between parallel lines of L36 L37
  measures "d229" distance of L38.start L38.end
  measures "d230" distance of L39.start L39.end
  measures "d231" angle of L40 L39
  measures "d232" distance of L41.start L41.end
  measures "d233" angle of L41 L42
  measures "d234" distance of L43.start L43.end
  measures "d235" distance of L44.start L44.end
  measures "d236" distance of L45.start L45.end
  measures "d237" distance of L46.start L46.end
  measures "d238" distance of L47.start L47.end
  measures "d239" diameter of A0
  measures "d240" diameter of A1
  measures "d241" diameter of A2
  measures "d242" diameter of A3
  measures "d243" diameter of A4
  measures "d244" diameter of A5
  measures "d245" diameter of A6
  measures "d246" diameter of A7
  measures "d247" diameter of A8
  measures "d248" diameter of A9
  measures "d249" diameter of A10
  measures "d250" distance of L48.start L48.end
  measures "d251" distance of L49.start L49.end
  measures "d252" diameter of A11
  measures "d253" diameter of A12
  measures "d257" distance of L50.start L50.end
  measures "d258" diameter of A13
extrude "拉伸41" add sketch "PCB草图" against normal blind 1.2 separate body contours L23 L22 L21 L20 L19 L18 L17 L16 L15 L14 L13 L12 | A3 L48 L39 | L39 L48 A3 | A4 L49 L41 | L41 L49 A4 | A0 | A1 | A2 | A5 | A6 | A7 | A8 | A9 | A10 | A11 | A12 | A13
ref_plane "pisition平面" through (0, 8.5, 0) normal (0, 1, 0) x (1, 0, 0)
sketch "position草图" plane through (0, 8.5, 0) normal (0, 1, 0) x (1, 0, 0)
  line L0 (-87.5, 137.5) -> (-87.5, -137.5)
  line L1 (-87.5, 137.5) -> (-87.5, 91)
  line L2 (51.5, 137.5) -> (-87.5, 137.5)
  line L3 (51.5, -137.5) -> (51.5, 137.5)
  line L4 (-87.5, -137.5) -> (51.5, -137.5)
  circle A0 centre (-80.4289, -44.4289) radius 1.5 projected
  circle A1 centre (-40.4289, -130.4289) radius 1.5 projected
  circle A2 centre (4.4289, -130.4289) radius 1.5 projected
  circle A3 centre (44.4289, -44.4289) radius 1.5 projected
  circle A4 centre (-18.0001, -44.4289) radius 1.5 projected
  circle A5 centre (-18.0001, 44.4289) radius 1.5 projected
  circle A6 centre (44.4289, 44.4289) radius 1.5 projected
  circle A7 centre (4.4289, 130.4289) radius 1.5 projected
  circle A8 centre (-40.4289, 130.4289) radius 1.5 projected
  circle A9 centre (-80.4289, 44.4289) radius 1.5 projected
  circle A10 centre (-55.3511, -132.7115) radius 1.5 projected
  circle A11 centre (-55.3511, -102.5115) radius 1.5 projected
  circle A12 centre (-26.8511, -132.7115) radius 1.5 projected
  circle A13 centre (-26.8511, -102.5115) radius 1.5 projected
  line L5 (-57.9261, -106.1115) -> (-51.4261, -106.1115) projected
  line L6 (-51.4261, -129.1115) -> (-57.9261, -129.1115) projected
  line L7 (-51.4261, -106.1115) -> (-51.4261, -129.1115) projected
  line L8 (-57.9261, -129.1115) -> (-57.9261, -106.1115) projected
  line L9 (-68.85, -137.15) -> (-68.85, -118.85) projected
  line L10 (-78, -128) -> (-78, -109) projected
  line L11 (-78, -109) -> (-78, -90) projected
  line L12 (-78, -90) -> (-78, -71) projected
  line L13 (-37.5518, -28.0147) -> (-47.2721, -48.8598) projected
  line L14 (-21.2884, -11.7513) -> (-37.5518, -28.0147) projected
  line L15 (-15.2859, 15.7913) -> (-33.6707, 34.176) projected
  line L16 (-33.6707, 34.176) -> (-44.6587, 57.74) projected
  line L17 (-44.6587, 57.74) -> (-46.9248, 83.6411) projected
  line L18 (-39.9237, 7.8713) -> (-58.3085, 26.2561) projected
  line L19 (-58.3085, 26.2561) -> (-69.2965, 49.8201) projected
  line L20 (-69.2965, 49.8201) -> (-71.5626, 75.7211) projected
  circle A14 centre (-47.2721, -48.8598) radius 10.5 projected
  circle A15 centre (-37.5518, -28.0147) radius 10.5 projected
  circle A16 centre (-21.2884, -11.7513) radius 10.5 projected
  circle A17 centre (-39.9237, 7.8713) radius 10.5 projected
  circle A18 centre (-15.2859, 15.7913) radius 10.5 projected
  circle A19 centre (-33.6707, 34.176) radius 10.5 projected
  circle A20 centre (-58.3085, 26.2561) radius 10.5 projected
  circle A21 centre (-65.0378, 1.142) radius 10.5 projected
  circle A22 centre (-69.2965, 49.8201) radius 10.5 projected
  circle A23 centre (-44.6587, 57.74) radius 10.5 projected
  circle A24 centre (-71.5626, 75.7211) radius 10.5 projected
  circle A25 centre (-46.9248, 83.6411) radius 10.5 projected
  circle A26 centre (29.1401, -6.9379) radius 13.5 projected
  circle A27 centre (21.9427, -33.997) radius 10.5 projected
  circle A28 centre (21.9427, 20.1213) radius 10.5 projected
  line L21 (-54.2971, -55.8848) -> (-40.2471, -55.8848)
  line L22 (-40.2471, -55.8848) -> (-40.2471, -41.8348)
  line L23 (-40.2471, -41.8348) -> (-54.2971, -41.8348)
  line L24 (-54.2971, -41.8348) -> (-54.2971, -55.8848)
  line L25 (-54.2971, -55.8848) -> (-40.2471, -41.8348) construction
  line L26 (-40.2471, -55.8848) -> (-54.2971, -41.8348) construction
  line L27 (-85.025, -135.025) -> (-70.975, -135.025)
  line L28 (-70.975, -135.025) -> (-70.975, -120.975)
  line L29 (-70.975, -120.975) -> (-85.025, -120.975)
  line L30 (-85.025, -120.975) -> (-85.025, -135.025)
  line L31 (-85.025, -135.025) -> (-70.975, -120.975) construction
  line L32 (-70.975, -135.025) -> (-85.025, -120.975) construction
  line L33 (-85.025, -116.025) -> (-70.975, -116.025)
  line L34 (-70.975, -116.025) -> (-70.975, -101.975)
  line L35 (-70.975, -101.975) -> (-85.025, -101.975)
  line L36 (-85.025, -101.975) -> (-85.025, -116.025)
  line L37 (-85.025, -116.025) -> (-70.975, -101.975) construction
  line L38 (-70.975, -116.025) -> (-85.025, -101.975) construction
  line L39 (-85.025, -97.025) -> (-70.975, -97.025)
  line L40 (-70.975, -97.025) -> (-70.975, -82.975)
  line L41 (-70.975, -82.975) -> (-85.025, -82.975)
  line L42 (-85.025, -82.975) -> (-85.025, -97.025)
  line L43 (-85.025, -97.025) -> (-70.975, -82.975) construction
  line L44 (-70.975, -97.025) -> (-85.025, -82.975) construction
  line L45 (-85.025, -78.025) -> (-70.975, -78.025)
  line L46 (-70.975, -78.025) -> (-70.975, -63.975)
  line L47 (-70.975, -63.975) -> (-85.025, -63.975)
  line L48 (-85.025, -63.975) -> (-85.025, -78.025)
  line L49 (-85.025, -78.025) -> (-70.975, -63.975) construction
  line L50 (-70.975, -78.025) -> (-85.025, -63.975) construction
  line L51 (-44.5768, -35.0397) -> (-30.5268, -35.0397)
  line L52 (-30.5268, -35.0397) -> (-30.5268, -20.9897)
  line L53 (-30.5268, -20.9897) -> (-44.5768, -20.9897)
  line L54 (-44.5768, -20.9897) -> (-44.5768, -35.0397)
  line L55 (-44.5768, -35.0397) -> (-30.5268, -20.9897) construction
  line L56 (-30.5268, -35.0397) -> (-44.5768, -20.9897) construction
  line L57 (-28.3134, -18.7763) -> (-14.2634, -18.7763)
  line L58 (-14.2634, -18.7763) -> (-14.2634, -4.7263)
  line L59 (-14.2634, -4.7263) -> (-28.3134, -4.7263)
  line L60 (-28.3134, -4.7263) -> (-28.3134, -18.7763)
  line L61 (-28.3134, -18.7763) -> (-14.2634, -4.7263) construction
  line L62 (-14.2634, -18.7763) -> (-28.3134, -4.7263) construction
  line L63 (-22.3109, 8.7663) -> (-8.2609, 8.7663)
  line L64 (-8.2609, 8.7663) -> (-8.2609, 22.8163)
  line L65 (-8.2609, 22.8163) -> (-22.3109, 22.8163)
  line L66 (-22.3109, 22.8163) -> (-22.3109, 8.7663)
  line L67 (-22.3109, 8.7663) -> (-8.2609, 22.8163) construction
  line L68 (-8.2609, 8.7663) -> (-22.3109, 22.8163) construction
  line L69 (-46.9487, 0.8463) -> (-32.8987, 0.8463)
  line L70 (-32.8987, 0.8463) -> (-32.8987, 14.8963)
  line L71 (-32.8987, 14.8963) -> (-46.9487, 14.8963)
  line L72 (-46.9487, 14.8963) -> (-46.9487, 0.8463)
  line L73 (-46.9487, 0.8463) -> (-32.8987, 14.8963) construction
  line L74 (-32.8987, 0.8463) -> (-46.9487, 14.8963) construction
  line L75 (-40.6957, 27.151) -> (-26.6457, 27.151)
  line L76 (-26.6457, 27.151) -> (-26.6457, 41.201)
  line L77 (-26.6457, 41.201) -> (-40.6957, 41.201)
  line L78 (-40.6957, 41.201) -> (-40.6957, 27.151)
  line L79 (-40.6957, 27.151) -> (-26.6457, 41.201) construction
  line L80 (-26.6457, 27.151) -> (-40.6957, 41.201) construction
  line L81 (-72.0628, -5.883) -> (-58.0128, -5.883)
  line L82 (-58.0128, -5.883) -> (-58.0128, 8.167)
  line L83 (-58.0128, 8.167) -> (-72.0628, 8.167)
  line L84 (-72.0628, 8.167) -> (-72.0628, -5.883)
  line L85 (-72.0628, -5.883) -> (-58.0128, 8.167) construction
  line L86 (-58.0128, -5.883) -> (-72.0628, 8.167) construction
  line L87 (-65.3335, 19.2311) -> (-51.2835, 19.2311)
  line L88 (-51.2835, 19.2311) -> (-51.2835, 33.2811)
  line L89 (-51.2835, 33.2811) -> (-65.3335, 33.2811)
  line L90 (-65.3335, 33.2811) -> (-65.3335, 19.2311)
  line L91 (-65.3335, 19.2311) -> (-51.2835, 33.2811) construction
  line L92 (-51.2835, 19.2311) -> (-65.3335, 33.2811) construction
  line L93 (-76.3215, 42.7951) -> (-62.2715, 42.7951)
  line L94 (-62.2715, 42.7951) -> (-62.2715, 56.8451)
  line L95 (-62.2715, 56.8451) -> (-76.3215, 56.8451)
  line L96 (-76.3215, 56.8451) -> (-76.3215, 42.7951)
  line L97 (-76.3215, 42.7951) -> (-62.2715, 56.8451) construction
  line L98 (-62.2715, 42.7951) -> (-76.3215, 56.8451) construction
  line L99 (-78.5876, 68.6961) -> (-64.5376, 68.6961)
  line L100 (-64.5376, 68.6961) -> (-64.5376, 82.7461)
  line L101 (-64.5376, 82.7461) -> (-78.5876, 82.7461)
  line L102 (-78.5876, 82.7461) -> (-78.5876, 68.6961)
  line L103 (-78.5876, 68.6961) -> (-64.5376, 82.7461) construction
  line L104 (-64.5376, 68.6961) -> (-78.5876, 82.7461) construction
  line L105 (-51.6837, 50.715) -> (-37.6337, 50.715)
  line L106 (-37.6337, 50.715) -> (-37.6337, 64.765)
  line L107 (-37.6337, 64.765) -> (-51.6837, 64.765)
  line L108 (-51.6837, 64.765) -> (-51.6837, 50.715)
  line L109 (-51.6837, 50.715) -> (-37.6337, 64.765) construction
  line L110 (-37.6337, 50.715) -> (-51.6837, 64.765) construction
  line L111 (-53.9498, 76.6161) -> (-39.8998, 76.6161)
  line L112 (-39.8998, 76.6161) -> (-39.8998, 90.6661)
  line L113 (-39.8998, 90.6661) -> (-53.9498, 90.6661)
  line L114 (-53.9498, 90.6661) -> (-53.9498, 76.6161)
  line L115 (-53.9498, 76.6161) -> (-39.8998, 90.6661) construction
  line L116 (-39.8998, 76.6161) -> (-53.9498, 90.6661) construction
  line L117 (14.9177, -41.022) -> (28.9677, -41.022)
  line L118 (28.9677, -41.022) -> (28.9677, -26.972)
  line L119 (28.9677, -26.972) -> (14.9177, -26.972)
  line L120 (14.9177, -26.972) -> (14.9177, -41.022)
  line L121 (14.9177, -41.022) -> (28.9677, -26.972) construction
  line L122 (28.9677, -41.022) -> (14.9177, -26.972) construction
  line L123 (21.9427, -13.9629) -> (35.9927, -13.9629)
  line L124 (35.9927, -13.9629) -> (35.9927, 0.0871)
  line L125 (35.9927, 0.0871) -> (21.9427, 0.0871)
  line L126 (21.9427, 0.0871) -> (21.9427, -13.9629)
  line L127 (21.9427, -13.9629) -> (35.9927, 0.0871) construction
  line L128 (35.9927, -13.9629) -> (21.9427, 0.0871) construction
  line L129 (14.9177, 13.2131) -> (28.9677, 13.2131)
  line L130 (28.9677, 13.2131) -> (28.9677, 27.2631)
  line L131 (28.9677, 27.2631) -> (14.9177, 27.2631)
  line L132 (14.9177, 27.2631) -> (14.9177, 13.2131)
  line L133 (14.9177, 13.2131) -> (28.9677, 27.2631) construction
  line L134 (28.9677, 13.2131) -> (14.9177, 27.2631) construction
  point P0 (0, 0)
  point P1 (28.9677, -6.9379)
  point P2 (21.9427, 20.2381)
  dimension "d317" = 14.05
  dimension "d318" = 14.05
  dimension "d319" = 14.05
  dimension "d320" = 14.05
  dimension "d321" = 14.05
  dimension "d322" = 14.05
  dimension "d323" = 14.05
  dimension "d324" = 14.05
  dimension "d325" = 14.05
  dimension "d326" = 14.05
  dimension "d327" = 14.05
  dimension "d328" = 14.05
  dimension "d329" = 14.05
  dimension "d330" = 14.05
  dimension "d331" = 14.05
  dimension "d332" = 14.05
  dimension "d333" = 14.05
  dimension "d334" = 14.05
  dimension "d335" = 14.05
  dimension "d336" = 14.05
  dimension "d337" = 14.05
  dimension "d338" = 14.05
  dimension "d339" = 14.05
  dimension "d340" = 14.05
  dimension "d341" = 14.05
  dimension "d342" = 14.05
  dimension "d343" = 14.05
  dimension "d344" = 14.05
  dimension "d345" = 14.05
  dimension "d346" = 14.05
  dimension "d347" = 14.05
  dimension "d348" = 14.05
  dimension "d349" = 14.05
  dimension "d350" = 14.05
  dimension "d351" = 14.05
  dimension "d352" = 14.05
  dimension "d353" = 14.05
  dimension "d354" = 14.05
  constraints: 238 end point, 38 midpoint
  measures "d317" distance of L23.end L22.end
  measures "d318" distance of L22.end L21.end
  measures "d319" distance of L29.end L28.end
  measures "d320" distance of L28.end L27.end
  measures "d321" distance of L35.end L34.end
  measures "d322" distance of L34.end L33.end
  measures "d323" distance of L41.end L40.end
  measures "d324" distance of L40.end L39.end
  measures "d325" distance of L47.end L46.end
  measures "d326" distance of L46.end L45.end
  measures "d327" distance of L53.end L52.end
  measures "d328" distance of L52.end L51.end
  measures "d329" distance of L59.end L58.end
  measures "d330" distance of L58.end L57.end
  measures "d331" distance of L65.end L64.end
  measures "d332" distance of L64.end L63.end
  measures "d333" distance of L71.end L70.end
  measures "d334" distance of L70.end L69.end
  measures "d335" distance of L77.end L76.end
  measures "d336" distance of L76.end L75.end
  measures "d337" distance of L83.end L82.end
  measures "d338" distance of L82.end L81.end
  measures "d339" distance of L89.end L88.end
  measures "d340" distance of L88.end L87.end
  measures "d341" distance of L95.end L94.end
  measures "d342" distance of L94.end L93.end
  measures "d343" distance of L101.end L100.end
  measures "d344" distance of L100.end L99.end
  measures "d345" distance of L107.end L106.end
  measures "d346" distance of L106.end L105.end
  measures "d347" distance of L113.end L112.end
  measures "d348" distance of L112.end L111.end
  measures "d349" distance of L119.end L118.end
  measures "d350" distance of L118.end L117.end
  measures "d351" distance of L125.end L124.end
  measures "d352" distance of L124.end L123.end
  measures "d353" distance of L131.end L130.end
  measures "d354" distance of L130.end L129.end
extrude "拉伸42" add sketch "position草图" against normal blind 1 separate body contours L2 L3 L4 L0 | A0 | A1 | A2 | A3 | A4 | A5 | A6 | A7 | A8 | A9 | A10 | A11 | A12 | A13 | L5 L7 L6 L8 | L33 L36 L35 L11 L10 | L10 L11 L35 L34 L33 | L39 L42 L41 L12 L11 | L11 L12 L41 L40 L39 | L14 L52 L51 L13 | L13 L51 L54 L53 L14 | L51 L52 L14 A15 L13 | L13 A15 L14 L53 L54 L51 | L75 L78 L77 L16 L15 | L76 L77 L16 A19 L15 | L15 A19 L16 L77 L78 L75 | L15 L16 L77 L76 | A23 L17 L107 L108 L105 L16 | L16 L105 L106 L107 L17 A23 | L105 L108 L107 L17 L16 | L16 L17 L107 L106 L105 | L87 L90 L89 L19 L18 | L88 L89 L19 A20 L18 | L18 A20 L19 L89 L90 L87 | L18 L19 L89 L88 | A22 L20 L95 L96 L93 L19 | L19 L93 L94 L95 L20 A22 | L93 L96 L95 L20 L19 | L19 L20 L95 L94 L93 | A14 | A16 | A17 | A18 | A21 | A24 | A25 | A26 | A27 | A28 | L24 L23 L22 L21 | L30 L29 L28 L27 | L48 L47 L46 L45 | L60 L59 L58 L57 | L66 L65 L64 L63 | L72 L71 L70 L69 | L84 L83 L82 L81 | L102 L101 L100 L99 | L114 L113 L112 L111 | L120 L119 L118 L117 | L126 L125 L124 L123 | L132 L131 L130 L129
sketch "底板PCB定位孔草图" plane through (0, -2, 0) normal (0, -1, 0) x (1, 0, 0)
  circle A0 centre (-80.4289, -44.4289) radius 1.5 projected
  circle A1 centre (-80.4289, 44.4289) radius 1.5 projected
  circle A2 centre (-40.4289, 130.4289) radius 1.5 projected
  circle A3 centre (4.4289, 130.4289) radius 1.5 projected
  circle A4 centre (44.4289, 44.4289) radius 1.5 projected
  circle A5 centre (44.4289, -44.4289) radius 1.5 projected
  circle A6 centre (-40.4289, -130.4289) radius 1.5 projected
  circle A7 centre (-93.9645, -65.5355) radius 1.5 projected
  circle A8 centre (-93.9645, -87.4645) radius 1.5 projected
  circle A9 centre (-93.9645, -10.9645) radius 1.5 projected
  circle A10 centre (-93.9645, 10.9645) radius 1.5 projected
  circle A11 centre (-18.0001, -44.4289) radius 1.5 projected
  circle A12 centre (-18.0001, 44.4289) radius 1.5 projected
  circle A13 centre (4.4289, -130.4289) radius 1.5 projected
  point P0 (0, 0)
hole "底板PCB定位孔" at (-40.4289, -2, -130.4289) at (-80.4289, -2, -44.4289) at (-18.0001, -2, -44.4289) at (44.4289, -2, -44.4289) at (44.4289, -2, 44.4289) at (-18.0001, -2, 44.4289) at (-80.4289, -2, 44.4289) at (-40.4289, -2, 130.4289) at (4.4289, -2, 130.4289) at (-93.9645, -2, -87.4645) at (-93.9645, -2, -65.5355) at (-93.9645, -2, -10.9645) at (-93.9645, -2, 10.9645) at (4.4289, -2, -130.4289) direction (0, 1, 0) diameter 2.7 end through all counterbore diameter 5.6 counterbore depth 1 bodies 1 6 7
hole "OLED定位孔" at (-55.3511, 8.5, 132.7115) at (-55.3511, 8.5, 102.5115) at (-26.8511, 8.5, 102.5115) at (-26.8511, 8.5, 132.7115) direction (0, -1, 0) diameter 3.2 end through all bodies 7
extrude "拉伸43" cut sketch "position草图" against normal through all contours L5 L7 L6 L8 bodies 7
extrude "拉伸44" cut sketch "position草图" against normal through all contours L33 L36 L35 L11 L10 | L10 L11 L35 L34 L33 | L39 L42 L41 L12 L11 | L11 L12 L41 L40 L39 | L14 L52 L51 L13 | L13 L51 L54 L53 L14 | L75 L78 L77 L16 L15 | L15 L16 L77 L76 | L105 L108 L107 L17 L16 | L16 L17 L107 L106 L105 | L87 L90 L89 L19 L18 | L18 L19 L89 L88 | L93 L96 L95 L20 L19 | L19 L20 L95 L94 L93 | L24 L23 L22 L21 | L30 L29 L28 L27 | L48 L47 L46 L45 | L60 L59 L58 L57 | L66 L65 L64 L63 | L72 L71 L70 L69 | L84 L83 L82 L81 | L102 L101 L100 L99 | L114 L113 L112 L111 | L120 L119 L118 L117 | L126 L125 L124 L123 | L132 L131 L130 L129 bodies 7
